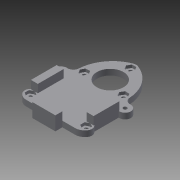
# Autodesk Inventor part: BallBearingHolderBottom
Saved by Autodesk Inventor 2015 (Build 190159000, 159)
## iProperties
Created: 2017-03-08
Part Number: BallBearingHolderBottom
Material: Generic
Document SubType Name: Modeling
Designer: Ernest
Density: 1 g/cm^3
Appearance: Default
Author: Ernest
Autodesk Inventor part; units mm, degrees
ref_plane "YZ Plane" through (0, 0, 0) normal (1, 0, 0) x (0, 1, 0)
ref_plane "XZ Plane" through (0, 0, 0) normal (0, 1, 0) x (-1, 0, 0)
ref_plane "XY Plane" through (0, 0, 0) normal (0, 0, 1) x (1, 0, 0)
sketch "Sketch1" plane through (0, 0, 0) normal (0, 0, 1) x (1, 0, 0)
  circle A0 centre (0, 0) radius 11.5
  line L0 (21.15, -51.53) -> (-21.15, -51.53) construction
  line L1 (-21.15, -51.53) -> (-21.15, -9.23) construction
  line L2 (-21.15, -9.23) -> (21.15, -9.23) construction
  line L3 (21.15, -9.23) -> (21.15, -51.53) construction
  circle A1 centre (0, 17.5) radius 1.6
  circle A2 centre (17, -5.5) radius 1.6
  circle A3 centre (-17, -5.5) radius 1.6
  line L4 (13.2517, -5.3162) -> (15.2851, -2.162)
  line L5 (15.2851, -2.162) -> (19.0333, -2.3458)
  line L6 (19.0333, -2.3458) -> (20.7483, -5.6838)
  line L7 (20.7483, -5.6838) -> (18.7149, -8.838)
  line L8 (18.7149, -8.838) -> (14.9667, -8.6542)
  line L9 (14.9667, -8.6542) -> (13.2517, -5.3162)
  line L10 (-14.9667, -8.6542) -> (-18.7149, -8.838)
  line L11 (-18.7149, -8.838) -> (-20.7483, -5.6838)
  line L12 (-20.7483, -5.6838) -> (-19.0333, -2.3458)
  line L13 (-19.0333, -2.3458) -> (-15.2851, -2.162)
  line L14 (-15.2851, -2.162) -> (-13.2517, -5.3162)
  line L15 (-13.2517, -5.3162) -> (-14.9667, -8.6542)
  line L16 (-1.8764, 14.25) -> (-3.7528, 17.5)
  line L17 (-3.7528, 17.5) -> (-1.8764, 20.75)
  line L18 (-1.8764, 20.75) -> (1.8764, 20.75)
  line L19 (1.8764, 20.75) -> (3.7528, 17.5)
  line L20 (3.7528, 17.5) -> (1.8764, 14.25)
  line L21 (1.8764, 14.25) -> (-1.8764, 14.25)
  line L22 (0, 0) -> (0, 17.5) construction
  line L23 (14.9667, -8.6542) -> (14.9667, -9.23) construction
  line L24 (13.2517, -5.3162) -> (12.7488, -5.0358) construction
  line L25 (21.15, -41.53) -> (27.15, -41.53)
  line L26 (27.15, -41.53) -> (27.15, -19.23)
  line L27 (27.15, -19.23) -> (21.15, -19.23)
  line L28 (21.15, -19.23) -> (21.15, -41.53)
  line L29 (-21.15, -41.53) -> (-27.15, -41.53)
  line L30 (-27.15, -41.53) -> (-27.15, -19.23)
  line L31 (-27.15, -19.23) -> (-21.15, -19.23)
  line L32 (-21.15, -19.23) -> (-21.15, -41.53)
  circle A4 centre (27.75, -14.88) radius 1.6
  circle A5 centre (-27.75, -14.88) radius 1.6
  line L33 (24.5, -16.7564) -> (24.5, -13.0036)
  line L34 (24.5, -13.0036) -> (27.75, -11.1272)
  line L35 (27.75, -11.1272) -> (31, -13.0036)
  line L36 (31, -13.0036) -> (31, -16.7564)
  line L37 (31, -16.7564) -> (27.75, -18.6328)
  line L38 (27.75, -18.6328) -> (24.5, -16.7564)
  line L39 (-27.75, -18.6328) -> (-31, -16.7564)
  line L40 (-31, -16.7564) -> (-31, -13.0036)
  line L41 (-31, -13.0036) -> (-27.75, -11.1272)
  line L42 (-27.75, -11.1272) -> (-24.5, -13.0036)
  line L43 (-24.5, -13.0036) -> (-24.5, -16.7564)
  line L44 (-24.5, -16.7564) -> (-27.75, -18.6328)
  circle A6 centre (-24.1, -44.9364) radius 1.6
  circle A7 centre (24.1, -44.9364) radius 1.6
  line L45 (-24.1, -48.6891) -> (-27.35, -46.8128)
  line L46 (-27.35, -46.8128) -> (-27.35, -43.06)
  line L47 (-27.35, -43.06) -> (-24.1, -41.1836)
  line L48 (-24.1, -41.1836) -> (-20.85, -43.06)
  line L49 (-20.85, -43.06) -> (-20.85, -46.8128)
  line L50 (-20.85, -46.8128) -> (-24.1, -48.6891)
  line L51 (24.1, -48.6891) -> (20.85, -46.8128)
  line L52 (20.85, -46.8128) -> (20.85, -43.06)
  line L53 (20.85, -43.06) -> (24.1, -41.1836)
  line L54 (24.1, -41.1836) -> (27.35, -43.06)
  line L55 (27.35, -43.06) -> (27.35, -46.8128)
  line L56 (27.35, -46.8128) -> (24.1, -48.6891)
  arc A8 (-27.3663, -9.8947) -> (-27.15, -19.8439) centre (-27.75, -14.88) ccw
  arc A9 (27.15, -19.8439) -> (27.3663, -9.8947) centre (27.75, -14.88) ccw
  arc A10 (-27.15, -40.9744) -> (-28.2818, -47.6773) centre (-24.1, -44.9364) ccw
  arc A11 (28.2818, -47.6773) -> (27.15, -40.9744) centre (24.1, -44.9364) ccw
  line L57 (21.15, -48.9734) -> (21.15, -51.53)
  line L58 (21.15, -51.53) -> (-21.15, -51.53)
  line L59 (-21.15, -51.53) -> (-21.15, -48.9734)
  arc A12 (1.7467, 22.185) -> (-1.7467, 22.185) centre (0, 17.5) ccw
  arc A13 (-27.3663, -9.8947) -> (-21.9913, -5.2047) centre (-26.9825, -4.9095) ccw
  arc A14 (21.9913, -5.2047) -> (27.3663, -9.8947) centre (26.9825, -4.9095) ccw
  arc A15 (21.15, -51.53) -> (28.2818, -47.6773) centre (21.15, -43.0028) ccw
  arc A16 (-28.2818, -47.6773) -> (-21.15, -51.53) centre (-21.15, -43.0028) ccw
  arc A17 (-1.7467, 22.185) -> (-21.9913, -5.2047) centre (9.1518, -7.047) ccw
  arc A18 (21.9913, -5.2047) -> (1.7467, 22.185) centre (-9.1518, -7.047) ccw
  dimension "d1" = 23
  dimension "d19" = 9.23
  dimension "d20" = 42.3
  dimension "d21" = 21.15
  dimension "d22" = 42.3
  dimension "d23" = 3.2
  dimension "d24" = 3.2
  dimension "d25" = 3.2
  dimension "d26" = 5.5
  dimension "d27" = 17
  dimension "d28" = 5.5
  dimension "d29" = 17
  dimension "d30" = 6.5
  dimension "d31" = 17.5
  dimension "d32" = 6.5
  dimension "d33" = 6.5
  dimension "d35" = 0.5758
  dimension "d36" = 0.5758
  dimension "d37" = 6
  dimension "d38" = 10
  dimension "d39" = 10
  dimension "d40" = 6
  dimension "d41" = 3.2
  dimension "d42" = 3.2
  dimension "d43" = 5.65
  dimension "d44" = 6.6
  dimension "d45" = 6.6
  dimension "d46" = 5.65
  dimension "d47" = 6.5
  dimension "d48" = 6.5
  dimension "d49" = 3.2
  dimension "d50" = 3.2
  dimension "d52" = 2.95
  dimension "d53" = 2.95
  dimension "d56" = 10
  dimension "d57" = 10
  dimension "d58" = 10
  dimension "d59" = 10
  dimension "d61" = 10
  dimension "d63" = 10
  dimension "d64" = 10
  dimension "d90" = 3.4064
  dimension "d91" = 3.4064
  dimension "d92" = 6.5
  dimension "d93" = 6.5
  constraints: 120 end point, 22 point on circle, 19 centre point, 14 coincident, 10 parallel, 10 tangent, 9 point on line, 6 perpendicular, 3 collinear, 3 horizontal, 1 equal length, 1 vertical, 91 other
  measures "d1" diameter of A0
  measures "d19" distance from line of point (0, 0) L2
  measures "d20" distance of L0.start L0.end
  measures "d21" distance from line of point (0, 0) L3
  measures "d22" distance of L2.end L0.start
  measures "d23" diameter of A2
  measures "d24" diameter of A1
  measures "d25" diameter of A3
  measures "d26" vertical distance of A2.centre point (0, 0)
  measures "d27" horizontal distance of point (0, 0) A2.centre
  measures "d28" vertical distance of point (0, 0) A3.centre
  measures "d29" horizontal distance of point (0, 0) A3.centre
  measures "d30" distance between parallel lines of L18 L21
  measures "d31" distance of point (0, 0) A1.centre
  measures "d32" distance between parallel lines of L5 L8
  measures "d33" distance between parallel lines of L13 L10
  measures "d35" distance of L8.end L23.end
  measures "d36" distance from line of L2 L10.start
  measures "d37" distance of L25.start L25.end
  measures "d38" distance between parallel lines of L2 L27
  measures "d39" distance between parallel lines of L25 L0
  measures "d40" distance of L29.start L29.end
  measures "d41" diameter of A5
  measures "d42" diameter of A4
  measures "d43" distance from line of L2 A4.centre
  measures "d44" distance from line of A4.centre L3
  measures "d45" distance from line of L1 A5.centre
  measures "d46" distance from line of L2 A5.centre
  measures "d47" distance between parallel lines of L44 L41
  measures "d48" distance between parallel lines of L34 L37
  measures "d49" diameter of A6
  measures "d50" diameter of A7
  measures "d52" distance from line of L1 A6.centre
  measures "d53" distance from line of L3 A7.centre
  measures "d56" diameter of A8
  measures "d57" diameter of A9
  measures "d58" diameter of A10
  measures "d59" diameter of A11
  measures "d61" diameter of A12
  measures "d63" diameter of A13
  measures "d64" diameter of A14
  measures "d90" distance from line of L29 A6.centre
  measures "d91" distance from line of L25 A7.centre
  measures "d92" distance between parallel lines of L49 L46
  measures "d93" distance between parallel lines of L52 L55
extrude "Extrusion5" add sketch "Sketch1" along normal blind 5 contours L25 L53 L52 L51 L56 L55 L54 L26 A11 A15 L58 A16 A10 L30 L29 L47 L46 L45 L50 L49 L48 L32 L31 A8 A13 A17 A12 A18 A14 A9 L27 L28 | L33 L34 L35 L36 L37 L38 | L39 L40 L41 L42 L43 L44
extrude "Extrusion6" add sketch "Sketch1" along normal blind 12 contours L28 L27 L26 L25 L54 L53 | L53 L54 L25 | L30 L31 L32 L29 L48 L47 | L47 L48 L29
extrude "Extrusion7" add sketch "Sketch1" along normal blind 2.5 contours L4 L5 L6 L7 L8 L9 | L10 L11 L12 L13 L14 L15 | L16 L17 L18 L19 L20 L21 | L53 L54 L25 | L25 L54 L55 L56 L51 L52 L53 | L47 L48 L29 | L29 L48 L49 L50 L45 L46 L47
extrude "Extrusion8" cut sketch "Sketch1" along normal blind 3 contours L33 L34 L35 L36 L37 L38 | L39 L40 L41 L42 L43 L44
sketch "Sketch2" plane through (0, 0, 5) normal (0, 0, 1) x (1, 0, 0)
  circle A0 centre (0, 17.5) radius 1.6 projected
  circle A1 centre (-17, -5.5) radius 1.6 projected
  circle A2 centre (-17, -5.5) radius 1.6 projected
  circle A3 centre (-24.1, -44.9364) radius 1.6 projected
  circle A4 centre (24.1, -44.9364) radius 1.6 projected
  circle A5 centre (24.1, -44.9364) radius 1.6 projected
  circle A6 centre (17, -5.5) radius 1.6 projected
  circle A7 centre (17, -5.5) radius 1.6 projected
  circle A8 centre (0, 0) radius 11.5 projected
  circle A9 centre (0, 0) radius 11.5 projected
  dimension "d77" = 23
  dimension "d78" = 17.5
  dimension "d79" = 34
  dimension "d80" = 5.5
  dimension "d81" = 48.2
  dimension "d82" = 44.9364
  measures "d77" diameter of A8
  measures "d78" distance of point (0, 0) A0.centre
  measures "d79" distance of A6.centre A1.centre
  measures "d80" vertical distance of point (0, 0) A1.centre
  measures "d81" distance of A4.centre A3.centre
  measures "d82" vertical distance of point (0, 0) A3.centre
sketch "Sketch3" plane through (0, 0, 5) normal (0, 0, 1) x (1, 0, 0)
  circle A0 centre (-27.75, -14.88) radius 1.6 projected
  circle A1 centre (27.75, -14.88) radius 1.6 projected
  circle A2 centre (0, 0) radius 11.5 projected
  line L0 (-3.7528, 17.5) -> (-1.8764, 20.75) projected
  line L1 (-1.8764, 20.75) -> (1.8764, 20.75) projected
  line L2 (1.8764, 20.75) -> (3.7528, 17.5) projected
  line L3 (3.7528, 17.5) -> (1.8764, 14.25) projected
  line L4 (1.8764, 14.25) -> (-1.8764, 14.25) projected
  line L5 (-1.8764, 14.25) -> (-3.7528, 17.5) projected
  line L6 (-18.7149, -8.838) -> (-20.7483, -5.6838) projected
  line L7 (-20.7483, -5.6838) -> (-19.0333, -2.3458) projected
  line L8 (-19.0333, -2.3458) -> (-15.2851, -2.162) projected
  line L9 (-15.2851, -2.162) -> (-13.2517, -5.3162) projected
  line L10 (-13.2517, -5.3162) -> (-14.9667, -8.6542) projected
  line L11 (-14.9667, -8.6542) -> (-18.7149, -8.838) projected
  line L12 (15.2851, -2.162) -> (19.0333, -2.3458) projected
  line L13 (19.0333, -2.3458) -> (20.7483, -5.6838) projected
  line L14 (20.7483, -5.6838) -> (18.7149, -8.838) projected
  line L15 (18.7149, -8.838) -> (14.9667, -8.6542) projected
  line L16 (14.9667, -8.6542) -> (13.2517, -5.3162) projected
  line L17 (13.2517, -5.3162) -> (15.2851, -2.162) projected
  arc A3 (21.15, -51.53) -> (28.2818, -47.6773) centre (21.15, -43.0028) ccw projected
  arc A4 (28.2818, -47.6773) -> (27.15, -40.9744) centre (24.1, -44.9364) ccw projected
  line L18 (27.15, -40.9744) -> (27.15, -41.53) projected
  line L19 (27.15, -41.53) -> (24.7, -41.53) projected
  line L20 (24.7, -41.53) -> (27.35, -43.06) projected
  line L21 (27.35, -43.06) -> (27.35, -46.8128) projected
  line L22 (27.35, -46.8128) -> (24.1, -48.6891) projected
  line L23 (24.1, -48.6891) -> (20.85, -46.8128) projected
  line L24 (20.85, -46.8128) -> (20.85, -43.06) projected
  line L25 (20.85, -43.06) -> (23.5, -41.53) projected
  line L26 (21.15, -41.53) -> (21.15, -19.23) projected
  line L27 (21.15, -19.23) -> (27.15, -19.23) projected
  line L28 (27.15, -19.23) -> (27.15, -19.8439) projected
  arc A5 (27.15, -19.8439) -> (27.3663, -9.8947) centre (27.75, -14.88) ccw projected
  arc A6 (21.9913, -5.2047) -> (27.3663, -9.8947) centre (26.9825, -4.9095) ccw projected
  arc A7 (21.9913, -5.2047) -> (1.7467, 22.185) centre (-9.1518, -7.047) ccw projected
  arc A8 (1.7467, 22.185) -> (-1.7467, 22.185) centre (0, 17.5) ccw projected
  arc A9 (-1.7467, 22.185) -> (-21.9913, -5.2047) centre (9.1518, -7.047) ccw projected
  arc A10 (-27.3663, -9.8947) -> (-21.9913, -5.2047) centre (-26.9825, -4.9095) ccw projected
  arc A11 (-27.3663, -9.8947) -> (-27.15, -19.8439) centre (-27.75, -14.88) ccw projected
  line L29 (-27.15, -19.8439) -> (-27.15, -19.23) projected
  line L30 (-27.15, -19.23) -> (-21.15, -19.23) projected
  line L31 (-21.15, -19.23) -> (-21.15, -41.53) projected
  line L32 (-24.7, -41.53) -> (-27.15, -41.53) projected
  line L33 (-23.5, -41.53) -> (-20.85, -43.06) projected
  line L34 (-20.85, -43.06) -> (-20.85, -46.8128) projected
  line L35 (-20.85, -46.8128) -> (-24.1, -48.6891) projected
  line L36 (-24.1, -48.6891) -> (-27.35, -46.8128) projected
  line L37 (-27.35, -46.8128) -> (-27.35, -43.06) projected
  line L38 (-27.35, -43.06) -> (-24.7, -41.53) projected
  line L39 (-27.15, -41.53) -> (-27.15, -40.9744) projected
  arc A12 (-27.15, -40.9744) -> (-28.2818, -47.6773) centre (-24.1, -44.9364) ccw projected
  arc A13 (-28.2818, -47.6773) -> (-21.15, -51.53) centre (-21.15, -43.0028) ccw projected
  line L40 (-21.15, -51.53) -> (21.15, -51.53) projected
  line L41 (-21.15, -51.53) -> (21.15, -51.53) projected
  line L42 (-10, -51.53) -> (10, -51.53)
  line L43 (10, -51.53) -> (10, -57.53)
  line L44 (10, -57.53) -> (-10, -57.53)
  line L45 (-10, -57.53) -> (-10, -51.53)
  line L46 (23.5, -41.53) -> (21.15, -41.53) projected
  line L47 (-21.15, -41.53) -> (-23.5, -41.53) projected
  dimension "d83" = 6
  dimension "d84" = 20
  dimension "d85" = 10
  constraints: 8 end point, 2 parallel, 1 horizontal, 1 perpendicular, 1 point on line
  measures "d83" distance of L44.end L42.start
  measures "d84" distance of L43.end L44.end
  measures "d85" distance from line of point (0, 0) L45
extrude "Extrusion9" add sketch "Sketch3" against normal blind 5 and the other way blind 7 contours L43 L44 L45 L40
equation "\"d21\" = 0.5 * d20"
equation "\"d22\" = d20"
body "Solid3"
